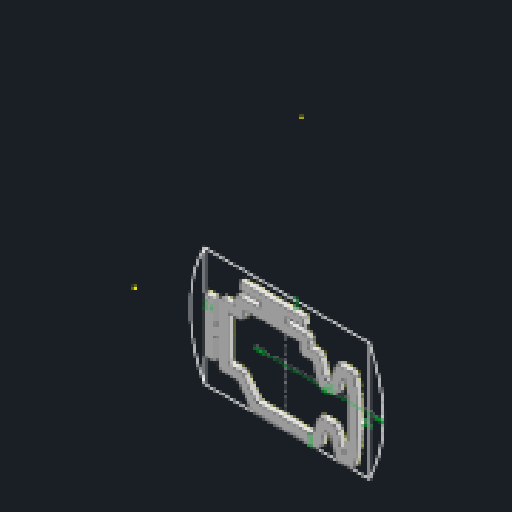
# Autodesk Inventor part: engine _light
Saved by Autodesk Inventor 2026 (Build 300175050, 175E)
## iProperties
Created: 2025-06-01
Part Number: engine _light
Material: Generic
Document SubType Name: Modeling
Designer: Natha
Density: 1 g/cm^3
Appearance: Default
Author: Natha
Autodesk Inventor part; units mm, degrees
ref_plane "YZ Plane" through (0, 0, 0) normal (1, 0, 0) x (0, 1, 0)
ref_plane "XZ Plane" through (0, 0, 0) normal (0, 1, 0) x (-1, 0, 0)
ref_plane "XY Plane" through (0, 0, 0) normal (0, 0, 1) x (1, 0, 0)
sketch "Sketch1" plane through (0, 0, 0) normal (0, 0, 1) x (1, 0, 0)
  circle A0 centre (-5.0359, -76.6135) radius 1.1 projected
  line L0 (-5.0359, -76.6135) -> (-5.0359, -51.6135) construction
  line L1 (-36.2859, -51.6135) -> (26.2141, -51.6135) construction
  line L2 (26.2141, -51.6135) -> (26.2141, -101.6135) construction
  line L3 (26.2141, -101.6135) -> (-36.2859, -101.6135) construction
  line L4 (-36.2859, -101.6135) -> (-36.2859, -51.6135) construction
  line L5 (-5.0359, -76.6135) -> (26.2141, -76.6135) construction
  line L6 (2.9641, -58.0535) -> (-19.6359, -58.0535)
  line L7 (-19.6359, -58.0535) -> (-19.6359, -60.8035)
  line L8 (-19.6359, -60.8035) -> (-12.7609, -60.8035)
  line L9 (-12.7609, -60.8035) -> (-12.7609, -62.6285)
  line L10 (-12.7609, -62.6285) -> (-19.6359, -62.6285)
  arc A1 (-19.6359, -62.6285) -> (-21.3019, -64.2945) centre (-19.6359, -64.2945) ccw
  line L11 (-19.6359, -60.8035) -> (-19.6359, -62.6285) construction
  line L12 (-21.3019, -66.1595) -> (-21.3019, -64.2945)
  line L13 (-21.3019, -66.1595) -> (-25.3019, -66.1595)
  arc A2 (-25.3019, -66.1595) -> (-26.9679, -67.8255) centre (-25.3019, -67.8255) ccw
  line L14 (-26.9679, -67.8255) -> (-26.9679, -75.6235)
  line L15 (-26.9679, -75.6235) -> (-28.3679, -75.6235)
  line L16 (-28.3679, -75.6235) -> (-28.3679, -67.8235)
  line L17 (-28.3679, -67.8235) -> (-31.7679, -67.8235)
  line L18 (-31.7679, -67.8235) -> (-31.7679, -86.8235)
  line L19 (-31.7679, -86.8235) -> (-28.3679, -86.8235)
  line L20 (-28.3679, -86.8235) -> (-28.3679, -79.0235)
  line L21 (-28.3679, -79.0235) -> (-26.9679, -79.0235)
  line L22 (-26.9679, -79.0235) -> (-26.9679, -86.8235)
  arc A3 (-26.9679, -86.8235) -> (-25.3019, -88.4895) centre (-25.3019, -86.8235) ccw
  line L23 (-25.3019, -88.4895) -> (-20.3359, -88.4895)
  line L24 (-20.3359, -88.4895) -> (-15.8208, -94.536)
  arc A4 (-15.8208, -94.536) -> (-14.6189, -95.1385) centre (-14.6189, -93.6385) ccw
  line L25 (-14.6189, -95.1385) -> (7.1805, -95.1385)
  arc A5 (7.1805, -95.1385) -> (8.784, -93.9247) centre (7.1805, -93.4725) ccw
  line L26 (8.784, -93.9247) -> (10.3101, -88.5135)
  line L27 (10.3101, -88.5135) -> (11.8101, -88.5135)
  line L28 (11.8101, -88.5135) -> (13.5395, -93.9985)
  arc A6 (13.5395, -93.9985) -> (15.1284, -95.1635) centre (15.1284, -93.4975) ccw
  line L29 (15.1284, -95.1635) -> (19.0084, -95.1635)
  arc A7 (19.0084, -95.1635) -> (20.6518, -93.771) centre (19.0084, -93.4975) ccw
  arc A8 (20.6518, -93.771) -> (20.6518, -67.5009) centre (-58.2626, -80.636) ccw
  line L30 (20.6518, -93.771) -> (20.6518, -67.5009) construction
  arc A9 (20.6518, -67.5009) -> (19.0143, -66.1135) centre (19.0143, -67.7735) ccw
  line L31 (19.0143, -66.1135) -> (15.1343, -66.1135)
  arc A10 (15.1343, -66.1135) -> (13.5454, -67.2785) centre (15.1343, -67.7795) ccw
  line L32 (13.5454, -67.2785) -> (11.816, -72.7635)
  line L33 (11.816, -72.7635) -> (10.316, -72.7635)
  line L34 (10.316, -72.7635) -> (8.7969, -67.3773)
  line L35 (2.9641, -58.0535) -> (3.0391, -58.0535)
  line L36 (3.0391, -58.0535) -> (3.0391, -60.8035)
  line L37 (3.0391, -60.8035) -> (-3.1109, -60.8035)
  line L38 (-3.1109, -60.8035) -> (-3.1109, -62.6285)
  line L39 (-3.1109, -62.6285) -> (3.0541, -62.6285)
  arc A11 (4.7141, -64.2885) -> (3.0541, -62.6285) centre (3.0541, -64.2885) ccw
  line L40 (4.7141, -64.2885) -> (4.7141, -66.1635)
  line L41 (4.7141, -66.1635) -> (7.1935, -66.1635)
  arc A12 (8.7969, -67.3773) -> (7.1935, -66.1635) centre (7.1935, -67.8295) ccw
  arc A13 (17.4947, -91.7285) -> (17.4954, -69.5485) centre (-58.2626, -80.636) ccw
  line L42 (17.4947, -91.7285) -> (16.4255, -91.7285)
  line L43 (16.4255, -91.7285) -> (14.3287, -85.0785)
  line L44 (14.3287, -85.0785) -> (7.7099, -85.0785)
  line L45 (7.7099, -85.0785) -> (5.8414, -91.7035)
  line L46 (5.8414, -91.7035) -> (-13.6489, -91.7035)
  line L47 (-13.6489, -91.7035) -> (-18.6139, -85.0545)
  line L48 (-18.6139, -85.0545) -> (-23.5329, -85.0545)
  line L49 (-23.5329, -85.0545) -> (-23.5329, -76.6135)
  line L50 (-23.5329, -76.6135) -> (-23.5329, -69.5945)
  line L51 (-23.5329, -69.5945) -> (-17.8669, -69.5945)
  line L52 (-17.8669, -69.5945) -> (-17.8669, -66.0635)
  line L53 (-17.8669, -66.0635) -> (-9.3259, -66.0635)
  line L54 (-9.3259, -66.0635) -> (-9.3259, -61.4885)
  line L55 (-9.3259, -61.4885) -> (-6.5459, -61.4885)
  line L56 (-6.5459, -61.4885) -> (-6.5459, -66.0635)
  line L57 (-6.5459, -66.0635) -> (1.2791, -66.0635)
  line L58 (1.2791, -66.0635) -> (1.2791, -69.5985)
  line L59 (1.2791, -69.5985) -> (5.8544, -69.5985)
  line L60 (5.8544, -69.5985) -> (7.7158, -76.1985)
  line L61 (7.7158, -76.1985) -> (14.3346, -76.1985)
  line L62 (14.3346, -76.1985) -> (16.4314, -69.5485)
  line L63 (16.4314, -69.5485) -> (17.4954, -69.5485)
  line L64 (-23.5329, -76.6135) -> (-5.0359, -76.6135) construction
  line L65 (-6.5459, -66.0635) -> (-9.3259, -66.0635)
  arc A14 (13.0515, -76.1985) -> (14.7205, -74.9747) centre (13.0515, -74.4485) ccw
  arc A15 (7.3562, -74.9235) -> (9.0405, -76.1985) centre (9.0405, -74.4485) ccw
  arc A16 (14.7146, -86.3022) -> (13.0456, -85.0785) centre (13.0456, -86.8285) ccw
  arc A17 (9.0346, -85.0785) -> (7.3503, -86.3535) centre (9.0346, -86.8285) ccw
  arc A18 (1.2791, -67.8485) -> (3.0291, -69.5985) centre (3.0291, -67.8485) ccw
  arc A19 (-19.6169, -69.5945) -> (-17.8669, -67.8445) centre (-19.6169, -67.8445) ccw
  arc A20 (-18.089, -85.7574) -> (-19.4912, -85.0545) centre (-19.4912, -86.8045) ccw
  point P0 (0, 0)
  dimension "d9" = 50
  dimension "d22" = 18.56
  dimension "d23" = 8
  dimension "d24" = 22.6
  dimension "d26" = 2.75
  dimension "d27" = 6.875
  dimension "d28" = 1.825
  dimension "d31" = 3.531
  dimension "d32" = 1.666
  dimension "d33" = 1.666
  dimension "d34" = 1.666
  dimension "d40" = 4
  dimension "d42" = 0.99
  dimension "d43" = 1.4
  dimension "d44" = 3.4
  dimension "d45" = 7.8
  dimension "d46" = 19
  dimension "d47" = 1.666
  dimension "d55" = 15.3
  dimension "d56" = 53.25
  dimension "d58" = 18.525
  dimension "d62" = 1.5
  dimension "d65" = 105.75
  dimension "d66" = 18
  dimension "d67" = 1.666
  dimension "d68" = 11.9
  dimension "d69" = 107.5
  dimension "d70" = 1.5
  dimension "d72" = 18.55
  dimension "d73" = 1.666
  dimension "d75" = 1.666
  dimension "d77" = 3.88
  dimension "d78" = 80
  dimension "d82" = 1.66
  dimension "d85" = 10.5
  dimension "d87" = 3.88
  dimension "d88" = 15.75
  dimension "d90" = 107.5
  dimension "d91" = 105.75
  dimension "d94" = 0.075
  dimension "d95" = 6.15
  dimension "d96" = 1.66
  dimension "d97" = 1.666
  dimension "d98" = 9.75
  dimension "d99" = 10.45
  dimension "d101" = 10.55
  dimension "d107" = 3.5
  dimension "d108" = 3.5
  dimension "d111" = 3.5
  dimension "d112" = 3.5
  dimension "d113" = 3.5
  dimension "d114" = 3.5
  dimension "d116" = 3.5
  constraints: 124 end point, 40 point on circle, 36 tangent, 20 centre point, 19 perpendicular, 17 point on line, 11 horizontal, 8 vertical, 5 equal length, 2 midpoint, 1 equal radius, 24 other
  measures "d9" distance of L1.end L2.end
  measures "d22" vertical distance of L0.start L6.start
  measures "d23" horizontal distance of L0.start L6.start
  measures "d24" distance of L6.start L6.end
  measures "d26" distance of L6.end L7.end
  measures "d27" distance of L7.end L8.end
  measures "d28" distance of L8.end L9.end
  measures "d31" vertical distance of L12.start L10.end
  measures "d32" horizontal distance of L10.end L12.start
  measures "d33" radius of A1
  measures "d34" radius of A2
  measures "d40" distance of L12.start L13.end
  measures "d42" vertical distance of L14.end L0.start
  measures "d43" distance of L14.end L15.end
  measures "d44" distance of L16.end L17.end
  measures "d45" distance of L15.end L16.end
  measures "d46" distance of L17.end L18.end
  measures "d47" radius of A3
  measures "d55" horizontal distance of L0.start L23.end
  measures "d56" angle of L23 L24
  measures "d58" distance from line of L0.start L25
  measures "d62" radius of A4
  measures "d65" angle of L25 L26
  measures "d66" distance from line of L0.start L26
  measures "d67" radius of A5
  measures "d68" distance from line of L0.start L27
  measures "d69" angle of L27 L28
  measures "d70" distance of L26.end L27.end
  measures "d72" distance from line of L0.start L29
  measures "d73" radius of A6
  measures "d75" radius of A7
  measures "d77" distance of L29.start L29.end
  measures "d78" radius of A8
  measures "d82" radius of A9
  measures "d85" distance from line of L0.start L31
  measures "d87" distance of L31.start L31.end
  measures "d88" distance between parallel lines of L27 L33
  measures "d90" angle of L33 L32
  measures "d91" angle of L34 L33
  measures "d94" distance of L6.start L35.end
  measures "d95" distance of L36.end L37.end
  measures "d96" radius of A11
  measures "d97" radius of A12
  measures "d98" distance from line of L0.start L40
  measures "d99" distance from line of L0.start L41
  measures "d101" distance from line of L0.start L57
  measures "d107" diameter of A14
  measures "d108" diameter of A15
  measures "d111" diameter of A16
  measures "d112" diameter of A17
  measures "d113" diameter of A18
  measures "d114" diameter of A19
  measures "d116" diameter of A20
extrude "Extrusion1" add sketch "Sketch1" along normal blind 2 contours L35 L36 L37 L38 L39 A11 L40 L41 A12 L34 L33 L32 A10 L31 A9 A8 A7 L29 A6 L28 L27 L26 A5 L25 A4 L24 L23 A3 L22 L21 L20 L19 L18 L17 L16 L15 L14 A2 L13 L12 A1 L10 L9 L8 L7 L6 | L65 L54 L55 L56
sketch "Sketch2" plane through (0, 0, 0) normal (0, 0, -1) x (-1, 0, 0)
  line L0 (-23.7374, -56.0535) -> (33.7679, -56.0535)
  line L1 (33.7679, -56.0535) -> (33.7679, -97.1385)
  line L2 (33.7679, -97.1385) -> (-23.7374, -97.1385)
  line L3 (-23.7374, -97.1385) -> (-23.7374, -56.0535)
  arc A0 (-23.7374, -56.0535) -> (-23.7374, -97.1385) centre (16.3001, -76.596) ccw
  line L4 (-3.0391, -58.0535) -> (19.6359, -58.0535) construction
  line L5 (-3.0391, -60.8035) -> (-3.0391, -58.0535) construction
  line L6 (3.1109, -60.8035) -> (-3.0391, -60.8035) construction
  line L7 (3.1109, -62.6285) -> (3.1109, -60.8035) construction
  line L8 (-3.0541, -62.6285) -> (3.1109, -62.6285) construction
  arc A1 (-3.0541, -62.6285) -> (-4.7141, -64.2885) centre (-3.0541, -64.2885) ccw construction
  line L9 (-4.7141, -66.1635) -> (-4.7141, -64.2885) construction
  line L10 (-7.1935, -66.1635) -> (-4.7141, -66.1635) construction
  arc A2 (-7.1935, -66.1635) -> (-8.7969, -67.3773) centre (-7.1935, -67.8295) ccw construction
  line L11 (-10.316, -72.7635) -> (-8.7969, -67.3773) construction
  line L12 (-11.816, -72.7635) -> (-10.316, -72.7635) construction
  line L13 (-13.5454, -67.2785) -> (-11.816, -72.7635) construction
  arc A3 (-13.5454, -67.2785) -> (-15.1343, -66.1135) centre (-15.1343, -67.7795) ccw construction
  line L14 (-19.0143, -66.1135) -> (-15.1343, -66.1135) construction
  arc A4 (-19.0143, -66.1135) -> (-20.6518, -67.5009) centre (-19.0143, -67.7735) ccw construction
  arc A5 (-20.6518, -67.5009) -> (-20.6518, -93.771) centre (58.2626, -80.636) ccw construction
  arc A6 (-20.6518, -93.771) -> (-19.0084, -95.1635) centre (-19.0084, -93.4975) ccw construction
  line L15 (-15.1284, -95.1635) -> (-19.0084, -95.1635) construction
  arc A7 (-15.1284, -95.1635) -> (-13.5395, -93.9985) centre (-15.1284, -93.4975) ccw construction
  line L16 (-11.8101, -88.5135) -> (-13.5395, -93.9985) construction
  line L17 (-10.3101, -88.5135) -> (-11.8101, -88.5135) construction
  line L18 (-8.784, -93.9247) -> (-10.3101, -88.5135) construction
  arc A8 (-8.784, -93.9247) -> (-7.1805, -95.1385) centre (-7.1805, -93.4725) ccw construction
  line L19 (14.6189, -95.1385) -> (-7.1805, -95.1385) construction
  arc A9 (14.6189, -95.1385) -> (15.8208, -94.536) centre (14.6189, -93.6385) ccw construction
  line L20 (20.3359, -88.4895) -> (15.8208, -94.536) construction
  line L21 (25.3019, -88.4895) -> (20.3359, -88.4895) construction
  arc A10 (25.3019, -88.4895) -> (26.9679, -86.8235) centre (25.3019, -86.8235) ccw construction
  line L22 (26.9679, -79.0235) -> (26.9679, -86.8235) construction
  line L23 (28.3679, -79.0235) -> (26.9679, -79.0235) construction
  line L24 (28.3679, -86.8235) -> (28.3679, -79.0235) construction
  line L25 (31.7679, -86.8235) -> (28.3679, -86.8235) construction
  line L26 (31.7679, -67.8235) -> (31.7679, -86.8235) construction
  line L27 (28.3679, -67.8235) -> (31.7679, -67.8235) construction
  line L28 (28.3679, -75.6235) -> (28.3679, -67.8235) construction
  line L29 (26.9679, -75.6235) -> (28.3679, -75.6235) construction
  line L30 (26.9679, -67.8255) -> (26.9679, -75.6235) construction
  arc A11 (26.9679, -67.8255) -> (25.3019, -66.1595) centre (25.3019, -67.8255) ccw construction
  line L31 (21.3019, -66.1595) -> (25.3019, -66.1595) construction
  line L32 (21.3019, -64.2945) -> (21.3019, -66.1595) construction
  arc A12 (21.3019, -64.2945) -> (19.6359, -62.6285) centre (19.6359, -64.2945) ccw construction
  line L33 (12.7609, -62.6285) -> (19.6359, -62.6285) construction
  line L34 (12.7609, -60.8035) -> (12.7609, -62.6285) construction
  line L35 (19.6359, -60.8035) -> (12.7609, -60.8035) construction
  line L36 (19.6359, -58.0535) -> (19.6359, -60.8035) construction
  line L37 (-17.4947, -91.7285) -> (-16.4255, -91.7285) construction
  arc A13 (-17.4954, -69.5485) -> (-17.4947, -91.7285) centre (58.2626, -80.636) ccw construction
  line L38 (-16.4314, -69.5485) -> (-17.4954, -69.5485) construction
  line L39 (-14.7205, -74.9747) -> (-16.4314, -69.5485) construction
  arc A14 (-14.7205, -74.9747) -> (-13.0515, -76.1985) centre (-13.0515, -74.4485) ccw construction
  line L40 (-9.0405, -76.1985) -> (-13.0515, -76.1985) construction
  arc A15 (-9.0405, -76.1985) -> (-7.3562, -74.9235) centre (-9.0405, -74.4485) ccw construction
  line L41 (-5.8544, -69.5985) -> (-7.3562, -74.9235) construction
  line L42 (-3.0291, -69.5985) -> (-5.8544, -69.5985) construction
  arc A16 (-3.0291, -69.5985) -> (-1.2791, -67.8485) centre (-3.0291, -67.8485) ccw construction
  line L43 (-1.2791, -66.0635) -> (-1.2791, -67.8485) construction
  line L44 (17.8669, -66.0635) -> (-1.2791, -66.0635) construction
  line L45 (17.8669, -67.8445) -> (17.8669, -66.0635) construction
  arc A17 (17.8669, -67.8445) -> (19.6169, -69.5945) centre (19.6169, -67.8445) ccw construction
  line L46 (23.5329, -69.5945) -> (19.6169, -69.5945) construction
  line L47 (23.5329, -85.0545) -> (23.5329, -69.5945) construction
  line L48 (19.4912, -85.0545) -> (23.5329, -85.0545) construction
  arc A18 (19.4912, -85.0545) -> (18.089, -85.7574) centre (19.4912, -86.8045) ccw construction
  line L49 (13.6489, -91.7035) -> (18.089, -85.7574) construction
  line L50 (-5.8414, -91.7035) -> (13.6489, -91.7035) construction
  line L51 (-7.3503, -86.3535) -> (-5.8414, -91.7035) construction
  arc A19 (-7.3503, -86.3535) -> (-9.0346, -85.0785) centre (-9.0346, -86.8285) ccw construction
  line L52 (-13.0456, -85.0785) -> (-9.0346, -85.0785) construction
  arc A20 (-13.0456, -85.0785) -> (-14.7146, -86.3022) centre (-13.0456, -86.8285) ccw construction
  line L53 (-16.4255, -91.7285) -> (-14.7146, -86.3022) construction
  arc A21 (-20.6518, -67.5009) -> (-20.6518, -93.771) centre (58.2626, -80.636) ccw construction
  line L54 (-21.7374, -80.636) -> (-18.3024, -80.6385) construction
  line L55 (16.3001, -76.596) -> (-28.6999, -76.596) construction
  line L56 (5.0152, -56.0535) -> (5.0152, -97.1385) construction
  arc A22 (33.7679, -97.1385) -> (33.7679, -56.0535) centre (-6.2696, -76.596) ccw
  circle A23 centre (5.0359, -76.6135) radius 1.1 projected
  point P0 (0, 0)
  dimension "d119" = 2
  dimension "d120" = 2
  dimension "d121" = 2
  dimension "d122" = 2
  dimension "d123" = 45
  constraints: 14 end point, 9 point on circle, 2 centre point, 2 midpoint, 2 parallel, 1 horizontal, 1 perpendicular, 1 symmetric about line, 1 other
  measures "d119" distance between parallel lines of L4 L0
  measures "d120" distance between parallel lines of L1 L26
  measures "d121" distance between parallel lines of L2 L19
  measures "d122" distance from line of L3 point (-21.737, -80.636)
  measures "d123" distance of L55.start L55.end
extrude "Extrusion2" add sketch "Sketch2" against normal blind 1
fillet "Fillet1" radius 10 4 edges at (23.7374, -97.1385, 0.5) (23.7374, -56.0535, 0.5) (-33.7679, -56.0535, 0.5) (-33.7679, -97.1385, 0.5)
body "Solid1"
